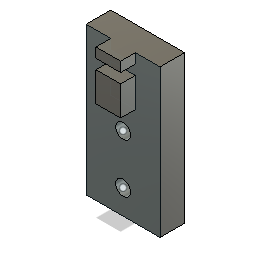
camera_back v2 (Autodesk Fusion 360 design; units mm, degrees)
Autodesk Fusion 360 part; units mm, degrees
sketch "Sketch1" plane through (0, 0, 0) normal (0, 0, 1) x (1, 0, 0)
  line L0 (0, 0) -> (15, 0)
  line L1 (15, 0) -> (15, 30)
  line L2 (15, 30) -> (0, 30)
  line L3 (0, 30) -> (0, 0)
  constraint horizontal L0
  constraint vertical L1
  constraint horizontal L2
  constraint vertical L3
  constraint coincident L0.start L3.end
extrude "Extrude1" add sketch "Sketch1" along normal blind 5
sketch "Sketch2" plane through (0, 0, 5) normal (0, 0, 1) x (1, 0, 0)
  line L0 (0, 30) -> (0, 0)
  line L1 (0, 0) -> (15, 0)
  line L2 (15, 0) -> (15, 30)
  line L3 (15, 30) -> (0, 30)
  line L4 (5, 30) -> (10, 30)
  line L5 (10, 30) -> (10, 20)
  line L6 (10, 20) -> (5, 20)
  line L7 (5, 20) -> (5, 30)
  dimension "d3" = 10
  constraint horizontal L4
  constraint vertical L5
  constraint horizontal L6
  constraint vertical L7
  constraint coincident L3 L4.start
  measures "d3" distance of L4.end L5.end
extrude "Extrude2" add sketch "Sketch2" along normal blind 3 contours L3 L4 L5 L6 L7
sketch "Sketch3" plane through (10, 0, 0) normal (1, 0, 0) x (0, 0, -1)
  line L0 (-5, 20) -> (-5, 30)
  line L1 (-5, 30) -> (-8, 30)
  line L2 (-8, 30) -> (-8, 20)
  line L3 (-8, 20) -> (-5, 20)
  line L4 (-8, 28) -> (-5, 28)
  line L5 (-5, 28) -> (-5, 26)
  line L6 (-5, 26) -> (-8, 26)
  line L7 (-8, 26) -> (-8, 28)
  dimension "d6" = 2
  dimension "d7" = 6
  constraint horizontal L4
  constraint vertical L5
  constraint horizontal L6
  constraint vertical L7
  constraint coincident L2 L4.start
  measures "d6" distance of L4.start L6.end
  measures "d7" distance of L3 L6
extrude "Extrude3" cut sketch "Sketch3" against normal blind 6 contours L0 L2 L4 L5 L6 L7
sketch "Sketch4" plane through (0, 0, 5) normal (0, 0, 1) x (1, 0, 0)
  line L0 (5, 28) -> (5, 30)
  line L1 (5, 30) -> (0, 30)
  line L2 (0, 30) -> (0, 0)
  line L3 (0, 0) -> (15, 0)
  line L4 (15, 0) -> (15, 30)
  line L5 (15, 30) -> (10, 30)
  line L6 (10, 30) -> (10, 28)
  line L7 (10, 28) -> (5, 28)
  line L8 (5, 26) -> (10, 26)
  line L9 (10, 26) -> (10, 20)
  line L10 (10, 20) -> (5, 20)
  line L11 (5, 20) -> (5, 26)
  point P0 (7.5, 5)
  point P1 (7.5, 15)
  dimension "d14" = 5
  dimension "d15" = 15
  measures "d14" distance of L3 P0
  measures "d15" distance of L3 P1
hole "Hole1" at (7.5, 5, 5) at (7.5, 15, 5) direction (0, 0, -1) diameter 3 end through all
